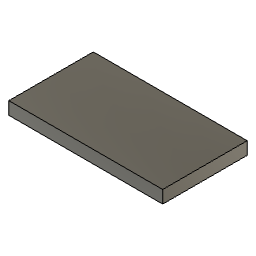
OpenBook Enclosure v2 (Autodesk Fusion 360 archive; units mm, degrees)
design "battery"
Autodesk Fusion 360 part; units mm, degrees
sketch "Sketch1" plane through (0, 0, 0) normal (0, 1, 0) x (1, 0, 0)
  line L0 (-50, 50) -> (26.5, 50)
  line L1 (26.5, 50) -> (26.5, 43.7)
  line L2 (26.5, 43.7) -> (-50, 43.7)
  line L3 (-50, 43.7) -> (-50, 50)
  dimension "d1" = 76.5
  dimension "d2" = 6.3
  constraint horizontal L0
  constraint vertical L1
  constraint horizontal L2
  constraint vertical L3
  measures "d1" distance of L0.start L0.end
  measures "d2" distance of L0.start L2.end
extrude "Extrude1" add sketch "Sketch1" along normal blind 42
